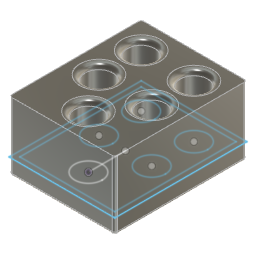
_3X2 light tester.ad88cc3c-a781-44f2-8fa2-05f255d4531a (Autodesk Fusion 360 design; units mm, degrees)
Autodesk Fusion 360 part; units mm, degrees
sketch "Sketch1" plane through (0, 0, 0) normal (0, 0, 1) x (1, 0, 0)
  circle A0 centre (0, 0) radius 2.6
  circle A1 centre (-5, 15) radius 2.6
  circle A2 centre (-5, 7) radius 2.6
  line L0 (0, 0) -> (0, 7)
  circle A3 centre (5, 7) radius 2.6
  circle A4 centre (5, 15) radius 2.6
  line L1 (-10, 20) -> (10, 20)
  line L2 (10, 20) -> (10, -5)
  line L3 (10, -5) -> (-10, -5)
  line L4 (-10, -5) -> (-10, 20)
  line L5 (-9, 19) -> (9, 19)
  line L6 (9, 19) -> (9, -4)
  line L7 (9, -4) -> (-9, -4)
  line L8 (-9, -4) -> (-9, 19)
  dimension "d1" = 5.2
  dimension "d2" = 5.2
  dimension "d3" = 5.2
  constraint coincident A0.centre L0.start
  constraint vertical L0
  constraint symmetric A1 L0 A4
  constraint symmetric A2 L0 A3
  constraint horizontal L1
  constraint vertical L2
  constraint horizontal L3
  constraint vertical L4
  constraint horizontal L5
  constraint vertical L6
  constraint horizontal L7
  constraint vertical L8
  measures "d1" diameter of A0
  measures "d2" diameter of A1
  measures "d3" diameter of A2
extrude "Extrude1" add sketch "Sketch1" along normal blind 10 contours L1 L2 L3 L4 | L5 L6 L7 L8
extrude "Extrude2" add sketch "Sketch1" against normal blind 3 contours L1 L2 L3 L4
fillet "Fillet1" radius 1 10 edges at (-7.4241, 15.9402, 10) (-7.4241, 7.9402, 10) (-2.4241, 0.9402, 10) (2.5759, 7.9402, 10) (2.5759, 15.9402, 10) (-7.4241, 15.9402, 0) (2.5759, 15.9402, 0) (2.5759, 7.9402, 0) (-7.4241, 7.9402, 0) (-2.4241, 0.9402, 0)
fillet "Fillet2" radius 0.5 7 edges at (-10, 20, 3.5) (-10, -5, 3.5) (0, -5, -3) (10, -5, 3.5) (10, 7.5, -3) (0, 20, -3) (10, 20, 3.5)
fillet "Fillet2" radius 0.5 1 edges at (-10, 7.5, -3)
